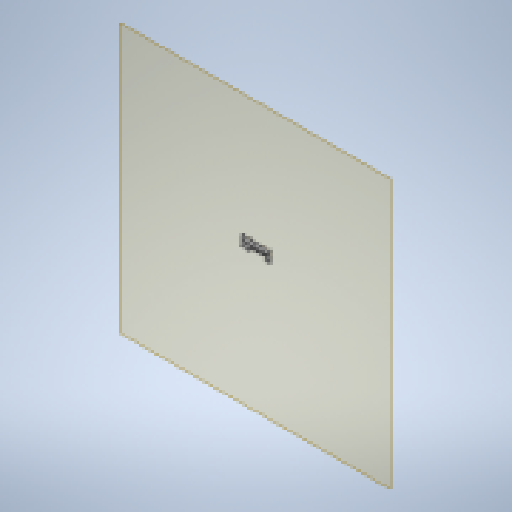
# Autodesk Inventor part: RobotStandHandle
Saved by Autodesk Inventor 2025.1 (Build 291241000, 241)
## iProperties
Created: 2026-05-10
Part Number: RobotStandHandle
Material: Generic
Document SubType Name: Modeling
Designer: User
Density: 1 g/cm^3
Appearance: Default
Author: User
## iProperties of the stored document RobotStandHandle_3DPrint.ipt
Created: 2026-05-11
Part Number: RobotStandHandle_3DPrint
Material: Generic
Document SubType Name: Modeling
Designer: User
Density: 1 g/cm^3
Appearance: Default
Author: User
Autodesk Inventor part; units mm, degrees
ref_plane "YZ Plane" through (0, 0, 0) normal (1, 0, 0) x (0, 1, 0)
ref_plane "XZ Plane" through (0, 0, 0) normal (0, 1, 0) x (-1, 0, 0)
ref_plane "Work Plane1" through (0, 0, 0) normal (0, 0, 1) x (1, 0, 0)
sketch "Sketch1" plane through (0, 0, 0) normal (0, 0, 1) x (1, 0, 0)
  line L0 (-7.7204, 28.6753) -> (4.2119, 28.6753) projected
  line L1 (4.2119, 28.6753) -> (4.2119, 0) projected
  line L2 (4.2119, 0) -> (34.2215, 0) projected
  line L3 (34.2215, 0) -> (34.2215, 72.9289) projected
  line L4 (34.2215, 72.9289) -> (-32.1076, 72.9289) projected
  line L5 (-32.1076, 72.9289) -> (-32.1076, 28.6753) projected
  line L6 (-32.1076, 28.6753) -> (-53.9396, 28.6753) projected
  line L7 (-53.9396, 28.6753) -> (-53.9396, 26.1753) projected
  line L8 (-7.7204, 26.1753) -> (-53.9396, 26.1753) projected
  line L9 (-7.7204, 26.1753) -> (-7.7204, 28.6753) projected
  line L10 (-111.3187, 26.1734) -> (-97.4187, 26.1734) projected
  line L11 (-97.4187, 26.1734) -> (-97.4187, 28.6734) projected
  line L12 (-119.2507, 28.6734) -> (-97.4187, 28.6734) projected
  line L13 (-119.2507, 28.6734) -> (-119.2507, 72.927) projected
  line L14 (-119.2507, 72.927) -> (-180.582, 72.927) projected
  line L15 (-180.582, 72.927) -> (-180.582, -0.0019) projected
  line L16 (-111.3187, -0.0019) -> (-180.582, -0.0019) projected
  line L17 (-111.3187, -0.0019) -> (-111.3187, 26.1734) projected
  line L18 (3.2119, -1) -> (3.2119, 27.6753)
  line L19 (3.2119, 27.6753) -> (-6.7204, 27.6753)
  line L20 (-6.7204, 27.6753) -> (-6.7204, 25.1753)
  line L21 (-8.7204, 25.1734) -> (-54.9377, 25.1734)
  line L22 (-33.1057, 73.927) -> (35.2196, 73.927)
  line L23 (35.2196, 73.927) -> (35.2196, -1)
  line L24 (35.2196, -1) -> (5.2119, -1)
  line L25 (-110.3187, 25.1734) -> (-96.4187, 25.1734)
  line L26 (-118.2507, 73.927) -> (-181.582, 73.927)
  line L27 (-181.582, 73.927) -> (-181.582, -1.0019)
  line L28 (-181.582, -1.0019) -> (-112.3187, -1.0019)
  line L29 (-110.3187, -1.0019) -> (-110.3187, 1)
  line L30 (5.2119, 1) -> (5.2119, 29.6753)
  line L31 (5.2119, 29.6753) -> (-8.7204, 29.6753)
  line L32 (-8.7204, 29.6753) -> (-8.7204, 27.1753)
  line L33 (-112.3187, 25.1734) -> (-112.3187, 0.9981)
  line L34 (5.2119, 1) -> (5.2119, -1)
  line L35 (-8.7204, 27.1753) -> (-8.7204, 25.0899)
  line L36 (-54.9377, 25.1734) -> (-96.4187, 25.1734)
  line L37 (-112.3187, 0.9981) -> (-112.3187, -1.0019)
  line L38 (-33.1057, 73.927) -> (-118.2507, 73.927)
  line L39 (-33.1057, 72.927) -> (-33.1057, 72.9289)
  line L40 (-118.2507, 29.6734) -> (-118.2507, 29.6753)
  line L41 (-107.1349, 25.1734) -> (-112.3187, 25.1734)
  point P0 (0, 0)
  dimension "d0" = 1
  dimension "d1" = 1
  dimension "d2" = 1
  constraints: 48 end point, 5 point on line, 3 perpendicular, 1 vertical, 6 other
  measures "d0" distance between parallel lines of L1 L18
  measures "d1" distance between parallel lines of L17 L29
  measures "d2" distance between parallel lines of L1 L30
extrude "Extrusion1" add sketch "Sketch1" along normal blind 4 contours L35 L21 L36 L25 L41 L17 L10 L11 L12 L13 L14 L15 L16 L37 L28 L27 L26 L38 L22 L23 L24 L34 L2 L3 L4 L5 L6 L7 L8 | L8 L7 L6 L5 L4 L3 L2 L34 L30 L31 L32 L35 | L41 L33 L37 L16 L15 L14 L13 L12 L11 L10 L17
sketch "Sketch2" plane through (-181.582, 73.927, 0) normal (0, 1, 0) x (1, 0, 0)
  line L0 (216.8016, 0) -> (0, 0) projected
  line L1 (0, 0) -> (0, -4) projected
  line L2 (216.8016, -4) -> (0, -4) projected
  line L3 (216.8016, 0) -> (216.8016, -4) projected
  line L4 (215.8035, 4.2425) -> (149.4744, 20.9053) projected
  line L5 (1, 3.518) -> (62.3312, 20.9233) projected
  line L6 (216.8016, -4) -> (0, -4)
  line L7 (0, -4) -> (0, 3)
  line L8 (0, 3) -> (216.8016, 3)
  line L9 (216.8016, 3) -> (216.8016, -4)
  point P0 (181.582, 0)
  point P1 (216.8016, 0)
  dimension "d6" = 7
  constraints: 8 end point, 2 parallel, 1 horizontal, 1 perpendicular
  measures "d6" distance of L6.end L7.end
extrude "Extrusion2" add sketch "Sketch2" along normal blind 4
sketch "Sketch3" plane through (5.2119, -1, 0) normal (0, -1, 0) x (1, 0, 0)
  line L0 (29.0097, -23.1331) -> (-1, -1) projected
  line L1 (0, 4) -> (30.0078, 4) projected
  line L2 (0, 0) -> (0, 4) projected
  line L3 (30.0078, 0) -> (30.0078, 4) projected
  line L4 (0, 0) -> (32.3681, -23.8725)
  line L5 (30.0078, 4) -> (30.0078, -22.1317)
  line L6 (30.0078, -3) -> (-186.7938, -3) projected
  point P0 (-5.2119, 0)
  point P1 (4.0676, -3)
  constraints: 4 end point, 2 point on line, 1 parallel
extrude "Extrusion3" add sketch "Sketch3" along normal blind 4 contours L1 L3 L5 L6 L4 L2
sketch "Sketch4" plane through (35.2196, 73.927, 0) normal (1, 0, 0) x (0, 0, -1)
  line L0 (3, -78.927) -> (-4, -78.927) projected
  line L1 (-4, 4) -> (3, 4) projected
  line L2 (3, 0) -> (3, 4) projected
  line L3 (-4, -78.927) -> (3, -78.927)
  line L4 (3, -78.927) -> (3, 4)
  line L5 (3, 4) -> (-4, 4)
  line L6 (-4, 4) -> (-4, -78.927)
  point P0 (0, -73.927)
  constraints: 8 end point, 2 parallel, 1 horizontal, 1 perpendicular
extrude "Extrusion4" add sketch "Sketch4" along normal blind 4
sketch "Sketch5" plane through (-181.582, -1.0019, 0) normal (-1, 0, 0) x (0, 0, 1)
  line L0 (-3, 78.9289) -> (4, 78.9289) projected
  line L1 (4, -3.9981) -> (0, -3.9981) projected
  line L2 (-3, 0.0019) -> (-3, -3.9981) projected
  line L3 (4, 78.9289) -> (-3, 78.9289)
  line L4 (-3, 78.9289) -> (-3, -3.9981)
  line L5 (-3, -3.9981) -> (4, -3.9981)
  line L6 (4, -3.9981) -> (4, 78.9289)
  line L7 (0, 0) -> (4, 0) projected
  line L8 (4, 0) -> (-3, 0.0019)
  point P0 (0, 1.0019)
  point P1 (-3, 78.9289)
  constraints: 10 end point, 2 parallel, 1 horizontal, 1 perpendicular
extrude "Extrusion5" add sketch "Sketch5" along normal blind 4 contours L0 L6 L7 L8 L4
sketch "Sketch6" plane through (-181.582, -1.0019, 0) normal (0, -1, 0) x (1, 0, 0)
  line L0 (36.2634, 6.688) -> (-2.5858, -21.9632) projected
  line L1 (-4, -3) -> (-4, 4) projected
  line L2 (0, -3) -> (-4, -3) projected
  line L3 (0, 4) -> (69.2633, 4) projected
  line L4 (-4, 4) -> (33.6504, 4)
  line L5 (33.6504, 4) -> (33.6504, -3)
  line L6 (33.6504, -3) -> (-4, -3)
  line L7 (-4, -3) -> (-4, 4)
  point P0 (181.582, 0)
  point P1 (23.1271, -3)
  point P2 (32.6186, 4)
  constraints: 8 end point, 2 parallel, 1 horizontal, 1 perpendicular
extrude "Extrusion6" add sketch "Sketch6" along normal blind 4 contours L0 L6 L2 L1 L4 L3
sketch "Sketch7" plane through (-181.582, -5.0019, 0) normal (0, -1, 0) x (1, 0, 0)
  line L0 (23.1271, -3) -> (32.6186, 4) projected
  line L1 (32.6186, 4) -> (-4, 4) projected
  line L2 (-4, 4) -> (-4, -3) projected
  line L3 (-4, -3) -> (23.1271, -3) projected
  line L4 (0, 4) -> (-4, 4) projected
  line L5 (0.7269, 4) -> (0.7269, -3)
  point P0 (181.582, 0)
  constraints: 2 end point, 2 point on line, 1 perpendicular
extrude "Extrusion7" add sketch "Sketch7" against normal blind 6 contours L3 L2 L1 L5
sketch "Sketch8" plane through (-181.582, 77.927, 0) normal (0, 1, 0) x (1, 0, 0)
  line L0 (-4, 3) -> (220.8016, 3) projected
  line L1 (215.8035, 4.2425) -> (149.4744, 20.9053) projected
  line L2 (1, 3.518) -> (62.3312, 20.9233) projected
  line L3 (1.4095, 2.075) -> (62.6358, 19.4505)
  line L4 (215.438, 2.7877) -> (149.1089, 19.4505)
  line L5 (149.1089, 19.4505) -> (62.6358, 19.4505)
  line L6 (149.1089, 19.4505) -> (62.6358, 19.4505)
  line L7 (62.6358, 19.4505) -> (62.6358, 3)
  line L8 (62.6358, 3) -> (149.1089, 3)
  line L9 (149.1089, 3) -> (149.1089, 19.4505)
  line L10 (105.8724, 19.4505) -> (105.8724, 3)
  line L11 (216.8016, 3) -> (0, 3) projected
  line L12 (93.3724, 3) -> (93.3724, 19.4505)
  line L13 (93.3724, 19.4505) -> (118.3724, 19.4505)
  line L14 (118.3724, 19.4505) -> (118.3724, 3)
  line L15 (118.3724, 3) -> (93.3724, 3)
  line L16 (93.3724, 3) -> (118.3724, 19.4505) construction
  line L17 (93.3724, 19.4505) -> (118.3724, 3) construction
  point P0 (181.582, 0)
  point P1 (105.8724, 11.2253)
  point P2 (62.6358, 19.4505)
  point P3 (4.669, 3)
  point P4 (214.593, 3)
  dimension "d19" = 1.5
  dimension "d20" = 1.5
  dimension "d21" = 25
  constraints: 28 end point, 6 parallel, 4 midpoint, 4 perpendicular, 2 horizontal, 2 point on line
  measures "d19" distance between parallel lines of L2 L3
  measures "d20" distance between parallel lines of L1 L4
  measures "d21" distance of L12.end L13.end
extrude "Extrusion8" add sketch "Sketch8" against normal blind 4 contours L0 L3 L7 | L9 L4 L0
fillet "Fillet1" radius 2 4 edges at (-32.473, 75.927, -3) (-118.9461, 75.927, -3) (-32.473, 75.927, -19.4505) (-118.9461, 75.927, -19.4505)
sketch "Sketch9" plane through (-181.582, 77.927, 0) normal (0, 1, 0) x (1, 0, 0)
  line L0 (80.9152, 12.1657) -> (62.6152, 12.1657) projected
  line L1 (62.6152, 37.4246) -> (62.6152, 19.9578) projected
  line L2 (80.9152, 10.1657) -> (62.6152, 10.1657)
  line L3 (60.6152, 37.4246) -> (60.6152, 19.9578)
  line L4 (62.6152, 10.1657) -> (55.3541, 10.1657)
  line L5 (60.6152, 19.9578) -> (60.6152, 10.1657)
  arc A0 (62.6358, 16.804) -> (60.0898, 18.728) centre (60.6358, 16.804) ccw projected
  line L6 (60.0898, 18.728) -> (4.669, 3) projected
  line L7 (-4, 3) -> (4.669, 3) projected
  line L8 (-4, -4) -> (-4, 3) projected
  line L9 (220.8016, -4) -> (-4, -4) projected
  line L10 (220.8016, 3) -> (220.8016, -4) projected
  line L11 (214.593, 3) -> (220.8016, 3) projected
  line L12 (214.593, 3) -> (151.5962, 18.8257) projected
  arc A1 (151.5962, 18.8257) -> (149.1089, 16.8859) centre (151.1089, 16.8859) ccw projected
  line L13 (149.1089, 16.8859) -> (149.1089, 5) projected
  arc A2 (147.1089, 3) -> (149.1089, 5) centre (147.1089, 5) ccw projected
  line L14 (64.6358, 3) -> (147.1089, 3) projected
  arc A3 (62.6358, 5) -> (64.6358, 3) centre (64.6358, 5) ccw projected
  line L15 (62.6358, 5) -> (62.6358, 16.804) projected
  point P0 (181.582, 0)
  point P1 (60.6152, 18.8039)
  point P2 (62.6358, 10.1657)
  dimension "d25" = 2
  dimension "d26" = 2
  constraints: 8 end point, 2 parallel, 1 horizontal, 1 perpendicular, 1 point on line
  measures "d25" distance between parallel lines of L0 L2
  measures "d26" distance between parallel lines of L1 L3
extrude "Extrusion9" cut sketch "Sketch9" against normal blind 4 contours L2 L4 L5 A0 L15
fillet "Fillet2" radius 2 2 edges at (-118.9461, 75.927, -10.1657) (-120.9667, 75.927, -18.8039)
fillet "Fillet3" radius 2 1 edges at (-120.9667, 75.927, -10.1657)
sketch "Sketch10" plane through (-185.582, -1.0019, 0) normal (-1, 0, 0) x (0, 0, 1)
  line L0 (-154.8556, -100.2785) -> (-154.8556, 111.7286) projected
  line L1 (-154.8556, 5.725) -> (5.0028, 5.725)
  line L2 (-3, 0.0019) -> (-3, 74.9289) projected
  line L3 (4, 78.9289) -> (4, -4) projected
  line L4 (4, 5.725) -> (9, 5.725)
  circle A0 centre (9, 5.725) radius 5
  circle A1 centre (9, 5.725) radius 2.5
  line L5 (9, 10.725) -> (4, 10.725)
  line L6 (9, 0.725) -> (4, 0.725)
  point P0 (0, 1.0019)
  dimension "d31" = 5
  dimension "d32" = 5
  constraints: 8 end point, 5 point on line, 3 point on circle, 2 centre point, 2 coincident, 2 perpendicular, 2 tangent, 1 midpoint, 1 parallel
  measures "d31" distance of L4.start L4.end
  measures "d32" diameter of A1
extrude "Extrusion10" add sketch "Sketch10" against normal blind 10
sketch "Sketch11" plane through (39.2196, 73.927, 0) normal (1, 0, 0) x (0, 0, -1)
  line L0 (-9, -74.2038) -> (-4, -74.2038) projected
  line L1 (-4, -64.2038) -> (-4, -74.2038) projected
  line L2 (-4, -64.2038) -> (-9, -64.2038) projected
  arc A0 (-9, -64.2038) -> (-9, -74.2038) centre (-9, -69.2038) ccw projected
  circle A1 centre (-9, -69.2038) radius 2.5 projected
  point P0 (0, -73.927)
extrude "Extrusion11" add sketch "Sketch11" against normal blind 10
sketch "Sketch12" plane through (-175.582, -1.0019, 0) normal (1, 0, 0) x (0, 0, -1)
  line L0 (-9, 0.725) -> (-4, 0.725) projected
  line L1 (-4, 10.725) -> (-4, 0.725) projected
  line L2 (-4, 10.725) -> (-9, 10.725) projected
  arc A0 (-9, 10.725) -> (-9, 0.725) centre (-9, 5.725) ccw projected
  circle A1 centre (-9, 5.725) radius 2.5 projected
  point P0 (0, 1.0019)
extrude "Extrusion12" add sketch "Sketch12" along normal up to surface (63.2633 mm away)
sketch "Sketch13" plane through (29.2196, 73.927, 0) normal (-1, 0, 0) x (0, 0, 1)
  arc A0 (9, -74.2038) -> (9, -64.2038) centre (9, -69.2038) ccw projected
  line L0 (9, -64.2038) -> (4, -64.2038) projected
  line L1 (4, -74.2038) -> (4, -64.2038) projected
  line L2 (4, -74.2038) -> (9, -74.2038) projected
  circle A1 centre (9, -69.2038) radius 2.5 projected
  point P0 (0, -73.927)
extrude "Extrusion13" add sketch "Sketch13" along normal up to surface (24.0078 mm away)
chamfer "Chamfer1" distance 4.72 angle 45 3 edges at (22.2158, 9.7232, 4) (22.2158, -0.2768, 4) (-148.9503, 9.7232, 4)
sketch "Sketch14" plane through (0, 0, 4) normal (0, 0, 1) x (1, 0, 0)
  line L0 (5.2119, 29.6753) -> (5.2119, 14.4432) projected
  line L1 (-8.7204, 29.6753) -> (5.2119, 29.6753) projected
  line L2 (-8.7204, 25.1734) -> (-8.7204, 29.6753) projected
  line L3 (-112.3187, 25.1734) -> (-8.7204, 25.1734) projected
  line L4 (-112.3187, 14.4432) -> (-112.3187, 25.1734) projected
  line L5 (-112.3187, 9.7232) -> (-112.3187, 14.4432) projected
  line L6 (5.2119, 14.4432) -> (5.2119, 9.7232) projected
  line L7 (9.2119, 9.7232) -> (9.2119, 14.4432)
  line L8 (9.2119, 14.4432) -> (9.2119, 33.6753)
  line L9 (9.2119, 33.6753) -> (-12.7204, 33.6753)
  line L10 (-12.7204, 33.6753) -> (-12.7204, 29.1734)
  line L11 (-12.7204, 29.1734) -> (-116.3187, 29.1734)
  line L12 (-116.3187, 29.1734) -> (-116.3187, 14.4432)
  line L13 (-116.3187, 14.4432) -> (-116.3187, 9.7232)
  line L14 (39.2196, 9.7232) -> (5.2119, 9.7232) projected
  line L15 (-185.582, 9.7232) -> (-112.3187, 9.7232) projected
  point P0 (0, 0)
  dimension "d44" = 4
  constraints: 14 end point, 6 other
  measures "d44" distance between parallel lines of L3 L11
extrude "Extrusion14" add sketch "Sketch14" along normal blind 4.5
sketch "Sketch15" plane through (5.2119, -5, 0) normal (0, -1, 0) x (1, 0, 0)
  line L0 (0, 4) -> (0, 0) projected
  line L1 (0, 0) -> (4.0676, -3) projected
  line L2 (4.0676, -3) -> (34.0078, -3) projected
  line L3 (34.0078, 4) -> (34.0078, -3) projected
  line L4 (0, 4) -> (34.0078, 4) projected
  line L5 (0, 0) -> (34.0078, -25.0819)
  line L6 (34.0078, -3) -> (34.0078, 4) projected
  line L7 (34.0078, -25.0819) -> (34.0078, 4)
  line L8 (34.0078, -3) -> (34.0078, -13)
  line L9 (34.0078, -13) -> (17.6263, -13)
  point P0 (-5.2119, 0)
  dimension "d47" = 10
  constraints: 8 end point, 2 point on line, 1 collinear, 1 perpendicular
  measures "d47" distance of L2.end L8.end
extrude "Extrusion15" add sketch "Sketch15" against normal up to surface (4 mm away) contours L2 L7 L9 L5
sketch "Sketch16" plane through (-181.582, 77.927, 0) normal (0, 1, 0) x (1, 0, 0)
  line L0 (220.8016, 3) -> (216.8016, 3) projected
  line L1 (220.8016, 13) -> (204.4202, 13) projected
  line L2 (220.8016, 3) -> (220.8016, -4) projected
  line L3 (220.8016, 3) -> (216.8016, 3)
  line L4 (216.8016, 3) -> (216.8016, 13)
  line L5 (216.8016, 13) -> (220.8016, 13)
  line L6 (220.8016, 13) -> (220.8016, 3)
  point P0 (181.582, 0)
  constraints: 8 end point, 2 parallel, 1 horizontal, 1 perpendicular, 1 point on line
extrude "Extrusion16" add sketch "Sketch16" against normal up to surface (78.927 mm away)
sketch "Sketch17" plane through (39.2196, 73.927, 0) normal (1, 0, 0) x (0, 0, -1)
  line L0 (17.7772, -66.5327) -> (3.5, -66.5327) projected
  line L1 (1.5, -68.5327) -> (3.5, -66.5327) projected
  line L2 (1.5, -68.5327) -> (19.7772, -68.5327) projected
  line L3 (17.7772, -66.5327) -> (19.7772, -68.5327) projected
  line L4 (19.7772, -68.5327) -> (19.7772, -41.6327) projected
  line L5 (17.7772, -43.6327) -> (19.7772, -41.6327) projected
  line L6 (17.7772, -43.6327) -> (17.7772, -66.5327) projected
  line L7 (17.7772, -66.5327) -> (19.7772, -68.5327) projected
  line L8 (3.5, -43.6327) -> (17.7772, -43.6327) projected
  line L9 (17.7772, -43.6327) -> (19.7772, -41.6327) projected
  line L10 (19.7772, -41.6327) -> (1.5, -41.6327) projected
  line L11 (1.5, -41.6327) -> (3.5, -43.6327) projected
  line L12 (1.5, -68.5327) -> (1.5, -41.6327)
  point P0 (0, -73.927)
  constraints: 2 end point, 1 vertical
extrude "Extrusion17" cut sketch "Sketch17" against normal blind 10
fillet "Fillet4" radius 2 4 edges at (37.2196, 5.3943, -13) (37.2196, 5.3943, -1.5) (37.2196, 32.2943, -1.5) (37.2196, 32.2943, -13)
sketch "Sketch18" plane through (-185.582, -1.0019, 0) normal (-1, 0, 0) x (0, 0, 1)
  line L0 (-3, 78.9289) -> (-3, -4) projected
  line L1 (-13, 78.9289) -> (-13, 35.2962) projected
  circle A0 centre (-15.218, 14.55) radius 8 projected
  circle A1 centre (-15.218, 36.2089) radius 8 projected
  circle A2 centre (-15.218, 58.1289) radius 8 projected
  arc A3 (-23.1511, 22.5971) -> (-23.1511, 6.5029) centre (-15.218, 14.55) ccw projected
  circle A4 centre (-15.218, 14.55) radius 11.3
  circle A5 centre (-15.218, 36.2089) radius 11.3
  circle A6 centre (-15.218, 58.1289) radius 11.3
  line L2 (0, -3.9981) -> (-13, -3.9981) projected
  line L3 (-13, -3.9981) -> (-13, 0.0019) projected
  line L4 (-3, 78.9289) -> (-13, 78.9289)
  line L5 (-13, 78.9289) -> (-13, -3.9981)
  line L6 (-13, -3.9981) -> (-3, -3.9981)
  line L7 (-3, -3.9981) -> (-3, 78.9289)
  line L8 (-15.218, 58.1289) -> (-7.218, 58.1289)
  line L9 (-1.5, 31.2962) -> (-1.5, 8.3962) projected
  line L10 (-7.218, 58.1289) -> (-7.218, 14.55)
  line L11 (-7.218, 14.55) -> (-7.218, 6.5694)
  line L12 (-7.218, 58.1289) -> (-7.218, 66.1095)
  point P0 (0, 1.0019)
  point P1 (-13, 69.2091)
  point P2 (-7.218, 50.1483)
  point P3 (-7.218, 44.1895)
  point P4 (-7.218, 28.2283)
  point P5 (-7.218, 22.5306)
  point P6 (-13, 3.4698)
  point P7 (-13, 0.0019)
  point P8 (-3, -3.9981)
  dimension "d56" = 22.6
  dimension "d55" = 22.6
  constraints: 16 end point, 3 coincident, 3 vertical, 2 horizontal alignment, 2 parallel, 2 perpendicular, 1 centre point, 1 horizontal, 1 point on line, 8 other
  measures "d55" diameter of A5
extrude "Extrusion18" add sketch "Sketch18" against normal blind 4 contours L0 L2 L3 L5 A4 L10 A5 A6 L1 L4
fillet "Fillet5" radius 2 6 edges at (-183.582, 49.1464, -7.218) (-183.582, 43.1876, -7.218) (-183.582, 27.2264, -7.218) (-183.582, 21.5287, -7.218) (-183.582, 2.4679, -13) (-183.582, 68.2072, -13)
sketch "Sketch19" plane through (-185.582, -1.0019, 0) normal (-1, 0, 0) x (0, 0, 1)
  line L0 (4, 78.9289) -> (4, 15.445) projected
  line L1 (8, 49.187) -> (0, 49.187)
  line L2 (0, 49.187) -> (0, 45.187)
  line L3 (0, 45.187) -> (8, 45.187)
  line L4 (8, 45.187) -> (8, 49.187)
  line L5 (8, 49.187) -> (0, 45.187) construction
  line L6 (0, 49.187) -> (8, 45.187) construction
  point P0 (0, 1.0019)
  point P1 (4, 47.187)
  point P2 (4, 49.187)
  point P3 (4, 45.187)
  dimension "d60" = 8
  dimension "d61" = 4
  constraints: 12 end point, 3 midpoint, 2 parallel, 1 horizontal, 1 perpendicular
  measures "d60" distance of L3.end L2.end
  measures "d61" distance of L2.end L1.end
extrude "Extrusion19" add sketch "Sketch19" against normal up to surface (224.8016 mm away) contours L1 L4 L3 L0
chamfer "Chamfer2" distance 2 angle 45 7 edges at (-73.1812, 48.1851, 4) (-73.1812, 44.1851, 4) (-116.3187, 21.8083, 4) (-64.5195, 29.1734, 4) (-12.7204, 31.4243, 4) (-1.7542, 33.6753, 4) (9.2119, 24.0592, 4)
chamfer "Chamfer3" distance 4 angle 45 2 edges at (-185.582, 46.1851, 8) (39.2196, 46.1851, 8)
sketch "Sketch20" plane through (-180.8551, -1.0019, 0) normal (1, 0, 0) x (0, 0, -1)
  line L0 (0, 0) -> (0, 2) projected
  line L1 (3, 0) -> (0, 0) projected
  line L2 (3, 0) -> (3, 2) projected
  line L3 (0, 2) -> (3, 2) projected
  point P0 (0, 1.0019)
extrude "Extrusion20" cut sketch "Sketch20" against normal up to surface (0.7269 mm away)
body "Solid1"
